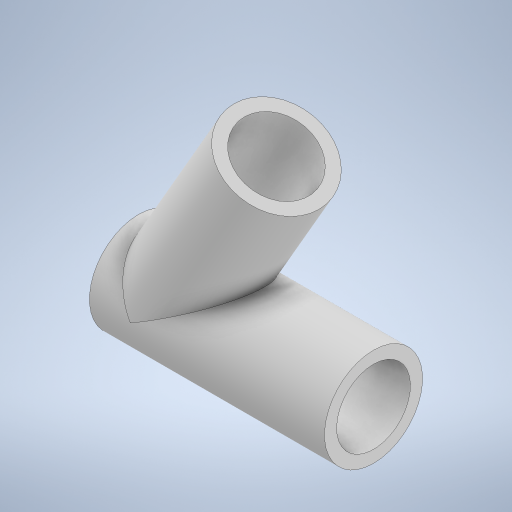
# Autodesk Inventor part: LAT-S24-SCH160-60
Saved by Autodesk Inventor 2023 (Build 270158000, 158)
## iProperties
Created: 2023-11-21
Part Number: LAT-S24-SCH160-60
Material: Generic
Document SubType Name: Modeling
Designer: Admin
Density: 1 g/cm^3
Appearance: Default
Author: Admin
Autodesk Inventor part; units mm, degrees
ref_plane "YZ Plane" through (0, 0, 0) normal (1, 0, 0) x (0, 1, 0)
ref_plane "XZ Plane" through (0, 0, 0) normal (0, 1, 0) x (-1, 0, 0)
sketch "Sweep Sketch" plane through (0, 0, 0) normal (0, 0, 1) x (1, 0, 0)
  line L0 (-730.25, 0) -> (730.25, 0)
  line L1 (-476.25, 0) -> (127, 1044.8596)
  point P0 (0, 0)
  point P1 (0, 0)
  dimension "B_Dimension" = 1206.5
  dimension "C_Dimension" = 254
  dimension "A_Dimension" = 1206.5
  dimension "angle" = 60
  constraints: 4 end point, 1 coincident, 1 horizontal, 1 midpoint, 1 point on line
  measures "B_Dimension" distance of L0.end L1.start
  measures "C_Dimension" distance of L0.start L1.start
  measures "A_Dimension" distance of L1.start L1.end
  measures "angle" angle of L0 L1
sketch "Base Tube Profile Sketch" plane through (0, 0, 0) normal (1, 0, 0) x (0, 1, 0)
  circle A0 centre (0, 0) radius 304.8
  circle A1 centre (0, 0) radius 229.3874
  dimension "baseOD" = 609.6
  dimension "wallThickness" = 75.4126
  constraints: 2 centre point, 2 coincident
  measures "baseOD" diameter of A0
  measures "wallThickness" radial gap between concentric circles of A0 A1
sweep "Sweep1" add profiles "Base Tube Profile Sketch" path "Sweep Sketch" path curves L0
ref_plane "Lateral Sketch Plane" through (127, 1044.8596, 0) normal (0.5, 0.8660254, 0) x (-0.8660254, 0.5, 0)
sketch "Lateral Tube Profile Sketch" plane through (127, 1044.8596, 0) normal (0.5, 0.8660254, 0) x (-0.8660254, 0.5, 0)
  circle A0 centre (0, 0) radius 304.8
  circle A1 centre (0, 0) radius 229.3874
  point P0 (-412.4446, 0)
  dimension "lateralOD" = 609.6
  dimension "lateralWallThickness" = 75.4126
  constraints: 2 centre point, 2 coincident
  measures "lateralOD" diameter of A0
  measures "lateralWallThickness" radial gap between concentric circles of A0 A1
extrude "Extrusion1" add sketch "Lateral Tube Profile Sketch" against normal up to surface
extrude "Extrusion2" cut sketch "Lateral Tube Profile Sketch" against normal up to surface contours A1 surface through (0, 0, 0) normal (0, 1, 0)
equation "\"lateralOD\" = baseOD"
equation "\"lateralWallThickness\" = wallThickness"
equation "\"nominalSize\" = 609.6"
body "Solid1"
